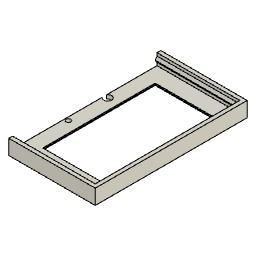
Solar Cell Case Bezel v14 (Autodesk Fusion 360 design; units mm, degrees)
Autodesk Fusion 360 part; units mm, degrees
sketch "Sketch1" plane through (0, 0, 0) normal (0, 0, 1) x (1, 0, 0)
  line L0 (0, 0) -> (44.2, 0)
  line L1 (44.2, 0) -> (44.2, 77.2)
  line L2 (44.2, 77.2) -> (0, 77.2)
  line L3 (0, 77.2) -> (0, 0)
  line L4 (0, 77.2) -> (0, 79.2)
  line L5 (0, 79.2) -> (46.2, 79.2)
  line L6 (46.2, 79.2) -> (46.2, -2)
  line L7 (46.2, -2) -> (0, -2)
  line L8 (0, -2) -> (0, 0)
  dimension "d1" = 44.2
  dimension "d2" = 77.2
  dimension "d3" = 2
  dimension "d4" = 46.2
  dimension "d5" = 2
  constraint horizontal L0
  constraint vertical L1
  constraint horizontal L2
  constraint vertical L3
  constraint coincident L0.start L3.end
  constraint perpendicular L2 L4
  constraint perpendicular L1 L5
  constraint perpendicular L5 L6
  constraint perpendicular L6 L7
  constraint perpendicular L0 L8
  measures "d1" distance of L0.start L0.end
  measures "d2" distance of L0.start L2.end
  measures "d3" distance of L2.end L4.end
  measures "d4" distance of L4.end L5.end
  measures "d5" distance of L0 L7
extrude "Extrude2" add sketch "Sketch1" along normal blind 8 contours L0 L1 L2 L4 L5 L6 L7 L8
extrude "Extrude1" add sketch "Sketch1" along normal blind 2 contours L0 L1 L2 L3
sketch "Sketch2" plane through (0, 0, 0) normal (-1, 0, 0) x (0, -1, 0)
  line L0 (-79.2, 0) -> (2, 0)
  line L1 (-77.2, 2) -> (-77.2, 8)
  line L2 (2, 8) -> (0, 8)
  line L3 (-79.2, 8) -> (-79.2, 0)
  line L4 (2, 0) -> (2, 8)
  line L5 (0, 8) -> (0, 2)
  line L6 (0, 2) -> (-77.2, 2)
  line L7 (-77.2, 8) -> (-79.2, 8)
  line L8 (-77.2, 3.55) -> (-76.2, 5)
  line L9 (-76.2, 5) -> (-77.2, 6.45)
  line L10 (-77.2, 3.55) -> (-77.2, 6.45)
  line L11 (0, 3.55) -> (-1, 5)
  line L12 (-1, 5) -> (0, 6.45)
  line L13 (0, 3.55) -> (0, 6.45)
  dimension "d10" = 5
  dimension "d11" = 2.9
  dimension "d12" = 1.55
  dimension "d13" = 1
  dimension "d14" = 1.45
  dimension "d15" = 1
  constraint coincident L1 L8.start
  constraint coincident L1 L9.end
  constraint parallel L1 L10
  constraint coincident L5 L11.start
  constraint coincident L5 L12.end
  constraint parallel L5 L13
  constraint horizontal L9.end L12.end
  constraint horizontal L8.start L11.start
  constraint horizontal L8.end L11.end
  measures "d11" distance of L8.start L9.end
  measures "d12" distance of L1.end L9.end
  measures "d13" distance of L8.end L10
  measures "d14" vertical distance of L8.end L9.end
  measures "d15" distance of L11.end L13
extrude "Extrude3" add sketch "Sketch2" against normal up to surface (44.2 mm away) contours L1 L8 L9 L10 | L5 L11 L12 L13
hole "Hole1" at (1.75, 28.1, 0) direction (0, 0, 1) diameter 2.5 depth 3 tip angle 118
hole "Hole2" at (1.75, 49.1, 0) direction (0, 0, 1) diameter 4.2 depth 3 tip angle 118
sketch "Sketch3" plane through (0, 0, 2) normal (0, 0, 1) x (-1, 0, 0)
  arc A0 (0, -47.9392) -> (0, -50.2608) centre (-1.75, -49.1) ccw
  line L0 (0, -47.9392) -> (0, 0)
  line L1 (0, 0) -> (-44.2, 0)
  line L2 (-44.2, 0) -> (-44.2, -77.2)
  line L3 (-44.2, -77.2) -> (0, -77.2)
  line L4 (0, -77.2) -> (0, -50.2608)
  circle A1 centre (-1.75, -28.1) radius 1.25
  line L5 (-7.6, -68.6) -> (-38.6, -68.6)
  line L6 (-38.6, -68.6) -> (-38.6, -8.6)
  line L7 (-38.6, -8.6) -> (-7.6, -8.6)
  line L8 (-7.6, -8.6) -> (-7.6, -68.6)
  line L9 (-44.2, 0) -> (-44.2, -77.2)
  line L10 (0, -76.2) -> (-44.2, -76.2)
  line L11 (0, -77.2) -> (0, 0)
  line L12 (-44.2, -77.2) -> (0, -77.2)
  dimension "d33" = 31
  dimension "d34" = 60
  dimension "d35" = 77.2
  dimension "d36" = 44.2
  dimension "d38" = 5.6
  dimension "d40" = 8.6
  constraint horizontal L5
  constraint vertical L6
  constraint horizontal L7
  constraint vertical L8
  measures "d33" distance of L5.start L5.end
  measures "d34" distance of L5.start L7.end
  measures "d35" distance of L1.end L2.end
  measures "d36" distance of L10.start L10.end
  measures "d38" distance of L6 L9
  measures "d40" distance of L5 L12
extrude "Extrude4" cut sketch "Sketch3" against normal blind 3 contours L5 L6 L7 L8
chamfer "Chamfer1" distance 1 angle 55 4 edges at (38.6, 38.6, 0) (23.1, 8.6, 0) (7.6, 38.6, 0) (23.1, 68.6, 0) measured on face at (17.9333, 1.5333, 0) measured on face at (17.9333, 1.5333, 0) measured on face at (17.9333, 1.5333, 0) measured on face at (17.9333, 1.5333, 0)
sketch "Sketch4" plane through (0, 0, 0) normal (0, 0, -1) x (1, 0, 0)
  circle A0 centre (1.75, -28.1) radius 1.25
  arc A1 (0, -50.2608) -> (0, -47.9392) centre (1.75, -49.1) ccw
  line L0 (0, -50.2608) -> (0, -79.2)
  line L1 (0, -79.2) -> (46.2, -79.2)
  line L2 (46.2, -79.2) -> (46.2, 2)
  line L3 (46.2, 2) -> (0, 2)
  line L4 (0, 2) -> (0, -47.9392)
  line L5 (39.6, -7.6) -> (39.6, -69.6)
  line L6 (39.6, -69.6) -> (6.6, -69.6)
  line L7 (6.6, -69.6) -> (6.6, -7.6)
  line L8 (6.6, -7.6) -> (39.6, -7.6)
  line L9 (40.9723, -71.136) -> (8.7716, -71.136) construction
  line L10 (8.7716, -71.136) -> (8.7716, -78.136) construction
  line L11 (8.7716, -78.136) -> (40.9723, -78.136) construction
  line L12 (40.9723, -78.136) -> (40.9723, -71.136) construction
  line L13 (7.9958, -5.6872) -> (37.8791, -5.6872) construction
  line L14 (37.8791, -5.6872) -> (37.8791, 1.3128) construction
  line L15 (37.8791, 1.3128) -> (7.9958, 1.3128) construction
  line L16 (7.9958, 1.3128) -> (7.9958, -5.6872) construction
  text T0 "Ferg Solar" font "Arial" height 7 align ink ink in box 0 x 0 at (40.9623, -71.156) x (-1, 0) y (0, -1) spacing 1 height is em
  text T1 "Go Green" font "Arial" height 7 align ink ink in box 0 x 0 at (8.0058, -5.6672) x (1, 0) y (0, 1) spacing 1 height is em
  constraint perpendicular L9 L10
  constraint parallel L9 L11
  constraint parallel L10 L12
  constraint perpendicular L13 L14
  constraint parallel L13 L15
  constraint parallel L14 L16
extrude "Extrude5" cut sketch "Sketch4" against normal blind 0.5 text T0 T1
sketch "Sketch5" plane through (0, 0, 0) normal (0, 0, -1) x (1, 0, 0)
  line L0 (39.6, -7.6) -> (39.6, -69.6)
  line L1 (39.6, -69.6) -> (6.6, -69.6)
  line L2 (6.6, -69.6) -> (6.6, -7.6)
  line L3 (6.6, -7.6) -> (39.6, -7.6)
  arc A0 (0, -50.2608) -> (0, -47.9392) centre (1.75, -49.1) ccw
  line L4 (0, -50.2608) -> (0, -79.2)
  line L5 (0, -79.2) -> (46.2, -79.2)
  line L6 (46.2, -79.2) -> (46.2, 2)
  line L7 (46.2, 2) -> (0, 2)
  line L8 (0, 2) -> (0, -47.9392)
  circle A1 centre (1.75, -28.1) radius 1.25
  line L9 (11.9912, -4.5495) -> (11.9912, -3.6164)
  line L10 (11.9912, -3.6164) -> (10.5181, -3.6164)
  line L11 (10.5181, -3.6164) -> (10.5181, -3.0285)
  line L12 (10.5181, -3.0285) -> (12.6406, -3.0251)
  line L13 (12.6406, -3.0251) -> (12.6406, -4.8845)
  spline S0 degree 3 poles (12.6406, -4.8845) (12.4792, -5.0053) (12.1657, -5.2398) (11.8065, -5.3953) (11.6323, -5.4707) knots 0 0 0 0 0.06025 0.116987 0.116987 0.116987 0.116987
  spline S1 degree 3 poles (11.6323, -5.4707) (11.4584, -5.528) (11.1118, -5.6422) (10.7474, -5.6589) (10.5659, -5.6672) knots 0 0 0 0 0.054662 0.108889 0.108889 0.108889 0.108889
  spline S2 degree 3 poles (10.5659, -5.6672) (10.3277, -5.6552) (9.861, -5.6316) (9.4336, -5.4432) (9.2244, -5.351) knots 0 0 0 0 0.070895 0.138867 0.138867 0.138867 0.138867
  spline S3 degree 3 poles (9.2244, -5.351) (9.0358, -5.2342) (8.6598, -5.0014) (8.4287, -4.6245) (8.3135, -4.4367) knots 0 0 0 0 0.065553 0.130667 0.130667 0.130667 0.130667
  spline S4 degree 3 poles (8.3135, -4.4367) (8.2238, -4.2287) (8.0399, -3.8022) (8.0174, -3.338) (8.0058, -3.1003) knots 0 0 0 0 0.06739 0.138134 0.138134 0.138134 0.138134
  spline S5 degree 3 poles (8.0058, -3.1003) (8.0181, -2.8616) (8.0423, -2.3889) (8.2225, -1.9514) (8.3118, -1.7348) knots 0 0 0 0 0.071122 0.140843 0.140843 0.140843 0.140843
  spline S6 degree 3 poles (8.3118, -1.7348) (8.4228, -1.5382) (8.6404, -1.153) (9.0106, -0.9114) (9.1919, -0.7932) knots 0 0 0 0 0.066656 0.130584 0.130584 0.130584 0.130584
  spline S7 degree 3 poles (9.1919, -0.7932) (9.3948, -0.7035) (9.8159, -0.5174) (10.2761, -0.4964) (10.5146, -0.4856) knots 0 0 0 0 0.065947 0.136861 0.136861 0.136861 0.136861
  spline S8 degree 3 poles (10.5146, -0.4856) (10.6886, -0.4918) (11.0247, -0.5038) (11.3435, -0.6103) (11.4973, -0.6616) knots 0 0 0 0 0.051926 0.10029 0.10029 0.10029 0.10029
  spline S9 degree 3 poles (11.4973, -0.6616) (11.6338, -0.7236) (11.8956, -0.8425) (12.092, -1.0519) (12.186, -1.1521) knots 0 0 0 0 0.044482 0.085284 0.085284 0.085284 0.085284
  spline S10 degree 3 poles (12.186, -1.1521) (12.2654, -1.2699) (12.4358, -1.5227) (12.5203, -1.8159) (12.5654, -1.9724) knots 0 0 0 0 0.042366 0.090875 0.090875 0.090875 0.090875
  line L14 (12.5654, -1.9724) -> (11.9673, -2.1364)
  spline S11 degree 3 poles (11.9673, -2.1364) (11.9305, -2.0199) (11.8633, -1.8069) (11.742, -1.6197) (11.687, -1.5349) knots 0 0 0 0 0.036444 0.066633 0.066633 0.066633 0.066633
  spline S12 degree 3 poles (11.687, -1.5349) (11.6227, -1.4646) (11.4868, -1.316) (11.3045, -1.2299) (11.2085, -1.1845) knots 0 0 0 0 0.028311 0.059812 0.059812 0.059812 0.059812
  spline S13 degree 3 poles (11.2085, -1.1845) (11.1002, -1.1462) (10.8769, -1.067) (10.64, -1.0577) (10.5181, -1.0529) knots 0 0 0 0 0.034265 0.070644 0.070644 0.070644 0.070644
  spline S14 degree 3 poles (10.5181, -1.0529) (10.3755, -1.0572) (10.1065, -1.0652) (9.8516, -1.151) (9.7319, -1.1914) knots 0 0 0 0 0.042524 0.080213 0.080213 0.080213 0.080213
  spline S15 degree 3 poles (9.7319, -1.1914) (9.6284, -1.2394) (9.4299, -1.3314) (9.2724, -1.4829) (9.197, -1.5554) knots 0 0 0 0 0.033966 0.065103 0.065103 0.065103 0.065103
  spline S16 degree 3 poles (9.197, -1.5554) (9.1332, -1.632) (9.0067, -1.7838) (8.9225, -1.9625) (8.8808, -2.051) knots 0 0 0 0 0.02978 0.059 0.059 0.059 0.059
  spline S17 degree 3 poles (8.8808, -2.051) (8.825, -2.211) (8.7111, -2.5374) (8.6968, -2.883) (8.6894, -3.0593) knots 0 0 0 0 0.050532 0.10313 0.10313 0.10313 0.10313
  spline S18 degree 3 poles (8.6894, -3.0593) (8.696, -3.2671) (8.7081, -3.6547) (8.853, -4.0138) (8.9202, -4.1804) knots 0 0 0 0 0.061793 0.115257 0.115257 0.115257 0.115257
  spline S19 degree 3 poles (8.9202, -4.1804) (9.0052, -4.3208) (9.1741, -4.5994) (9.4533, -4.7671) (9.5918, -4.8503) knots 0 0 0 0 0.04845 0.096145 0.096145 0.096145 0.096145
  spline S20 degree 3 poles (9.5918, -4.8503) (9.7412, -4.9141) (10.0405, -5.0419) (10.3655, -5.06) (10.5283, -5.0691) knots 0 0 0 0 0.048329 0.096832 0.096832 0.096832 0.096832
  spline S21 degree 3 poles (10.5283, -5.0691) (10.6715, -5.062) (10.9598, -5.0477) (11.2321, -4.9516) (11.3691, -4.9033) knots 0 0 0 0 0.042755 0.086105 0.086105 0.086105 0.086105
  spline S22 degree 3 poles (11.3691, -4.9033) (11.4924, -4.8515) (11.7141, -4.7583) (11.906, -4.6137) (11.9912, -4.5495) knots 0 0 0 0 0.039923 0.071805 0.071805 0.071805 0.071805
  line L15 (23.2739, -4.5495) -> (23.2739, -3.6164)
  line L16 (23.2739, -3.6164) -> (21.8008, -3.6164)
  line L17 (21.8008, -3.6164) -> (21.8008, -3.0285)
  line L18 (21.8008, -3.0285) -> (23.9233, -3.0251)
  line L19 (23.9233, -3.0251) -> (23.9233, -4.8845)
  spline S23 degree 3 poles (23.9233, -4.8845) (23.7619, -5.0053) (23.4484, -5.2398) (23.0892, -5.3953) (22.915, -5.4707) knots 0 0 0 0 0.06025 0.116987 0.116987 0.116987 0.116987
  spline S24 degree 3 poles (22.915, -5.4707) (22.7411, -5.528) (22.3946, -5.6422) (22.0301, -5.6589) (21.8486, -5.6672) knots 0 0 0 0 0.054662 0.108889 0.108889 0.108889 0.108889
  spline S25 degree 3 poles (21.8486, -5.6672) (21.6104, -5.6552) (21.1437, -5.6316) (20.7163, -5.4432) (20.5071, -5.351) knots 0 0 0 0 0.070895 0.138867 0.138867 0.138867 0.138867
  spline S26 degree 3 poles (20.5071, -5.351) (20.3185, -5.2342) (19.9425, -5.0014) (19.7114, -4.6245) (19.5962, -4.4367) knots 0 0 0 0 0.065553 0.130667 0.130667 0.130667 0.130667
  spline S27 degree 3 poles (19.5962, -4.4367) (19.5065, -4.2287) (19.3226, -3.8022) (19.3001, -3.338) (19.2886, -3.1003) knots 0 0 0 0 0.06739 0.138134 0.138134 0.138134 0.138134
  spline S28 degree 3 poles (19.2886, -3.1003) (19.3008, -2.8616) (19.325, -2.3889) (19.5053, -1.9514) (19.5945, -1.7348) knots 0 0 0 0 0.071122 0.140843 0.140843 0.140843 0.140843
  spline S29 degree 3 poles (19.5945, -1.7348) (19.7055, -1.5382) (19.9232, -1.153) (20.2934, -0.9114) (20.4746, -0.7932) knots 0 0 0 0 0.066656 0.130584 0.130584 0.130584 0.130584
  spline S30 degree 3 poles (20.4746, -0.7932) (20.6775, -0.7035) (21.0986, -0.5174) (21.5589, -0.4964) (21.7974, -0.4856) knots 0 0 0 0 0.065947 0.136861 0.136861 0.136861 0.136861
  spline S31 degree 3 poles (21.7974, -0.4856) (21.9714, -0.4918) (22.3074, -0.5038) (22.6263, -0.6103) (22.78, -0.6616) knots 0 0 0 0 0.051926 0.10029 0.10029 0.10029 0.10029
  spline S32 degree 3 poles (22.78, -0.6616) (22.9165, -0.7236) (23.1783, -0.8425) (23.3747, -1.0519) (23.4687, -1.1521) knots 0 0 0 0 0.044482 0.085284 0.085284 0.085284 0.085284
  spline S33 degree 3 poles (23.4687, -1.1521) (23.5482, -1.2699) (23.7185, -1.5227) (23.803, -1.8159) (23.8481, -1.9724) knots 0 0 0 0 0.042366 0.090874 0.090874 0.090874 0.090874
  line L20 (23.8481, -1.9724) -> (23.25, -2.1364)
  spline S34 degree 3 poles (23.25, -2.1364) (23.2132, -2.0199) (23.146, -1.8069) (23.0247, -1.6197) (22.9697, -1.5349) knots 0 0 0 0 0.036444 0.066633 0.066633 0.066633 0.066633
  spline S35 degree 3 poles (22.9697, -1.5349) (22.9054, -1.4646) (22.7695, -1.316) (22.5872, -1.2299) (22.4912, -1.1845) knots 0 0 0 0 0.028311 0.059812 0.059812 0.059812 0.059812
  spline S36 degree 3 poles (22.4912, -1.1845) (22.3829, -1.1462) (22.1596, -1.067) (21.9227, -1.0577) (21.8008, -1.0529) knots 0 0 0 0 0.034265 0.070644 0.070644 0.070644 0.070644
  spline S37 degree 3 poles (21.8008, -1.0529) (21.6582, -1.0572) (21.3892, -1.0652) (21.1344, -1.151) (21.0146, -1.1914) knots 0 0 0 0 0.042524 0.080213 0.080213 0.080213 0.080213
  spline S38 degree 3 poles (21.0146, -1.1914) (20.9111, -1.2394) (20.7126, -1.3314) (20.5551, -1.4829) (20.4797, -1.5554) knots 0 0 0 0 0.033966 0.065103 0.065103 0.065103 0.065103
  spline S39 degree 3 poles (20.4797, -1.5554) (20.4159, -1.632) (20.2894, -1.7838) (20.2053, -1.9625) (20.1636, -2.051) knots 0 0 0 0 0.02978 0.059 0.059 0.059 0.059
  spline S40 degree 3 poles (20.1636, -2.051) (20.1077, -2.211) (19.9938, -2.5374) (19.9795, -2.883) (19.9722, -3.0593) knots 0 0 0 0 0.050532 0.10313 0.10313 0.10313 0.10313
  spline S41 degree 3 poles (19.9722, -3.0593) (19.9787, -3.2671) (19.9908, -3.6547) (20.1357, -4.0138) (20.2029, -4.1804) knots 0 0 0 0 0.061793 0.115257 0.115257 0.115257 0.115257
  spline S42 degree 3 poles (20.2029, -4.1804) (20.2879, -4.3208) (20.4568, -4.5994) (20.736, -4.7671) (20.8745, -4.8503) knots 0 0 0 0 0.04845 0.096145 0.096145 0.096145 0.096145
  spline S43 degree 3 poles (20.8745, -4.8503) (21.0239, -4.9141) (21.3232, -5.0419) (21.6482, -5.06) (21.811, -5.0691) knots 0 0 0 0 0.048329 0.096832 0.096832 0.096832 0.096832
  spline S44 degree 3 poles (21.811, -5.0691) (21.9542, -5.062) (22.2425, -5.0477) (22.5148, -4.9516) (22.6518, -4.9033) knots 0 0 0 0 0.042755 0.086104 0.086104 0.086104 0.086104
  spline S45 degree 3 poles (22.6518, -4.9033) (22.7751, -4.8515) (22.9968, -4.7583) (23.1887, -4.6137) (23.2739, -4.5495) knots 0 0 0 0 0.039923 0.071805 0.071805 0.071805 0.071805
  line L21 (25.4307, -3.6814) -> (25.4307, -5.5817)
  line L22 (25.4307, -5.5817) -> (24.8154, -5.5817)
  line L23 (24.8154, -5.5817) -> (24.8154, -1.9519)
  line L24 (24.8154, -1.9519) -> (25.3691, -1.9519)
  line L25 (25.3691, -1.9519) -> (25.3691, -2.5022)
  spline S46 degree 3 poles (25.3691, -2.5022) (25.4308, -2.3903) (25.5357, -2.2002) (25.6949, -2.0534) (25.7605, -1.9929) knots 0 0 0 0 0.037975 0.064591 0.064591 0.064591 0.064591
  spline S47 degree 3 poles (25.7605, -1.9929) (25.8217, -1.957) (25.9438, -1.8854) (26.0849, -1.875) (26.1553, -1.8698) knots 0 0 0 0 0.02098 0.041844 0.041844 0.041844 0.041844
  spline S48 degree 3 poles (26.1553, -1.8698) (26.2618, -1.8797) (26.4865, -1.9004) (26.6839, -2.0103) (26.7876, -2.0681) knots 0 0 0 0 0.031749 0.066919 0.066919 0.066919 0.066919
  line L26 (26.7876, -2.0681) -> (26.5757, -2.6389)
  spline S49 degree 3 poles (26.5757, -2.6389) (26.5021, -2.6) (26.3605, -2.5252) (26.2011, -2.512) (26.1245, -2.5056) knots 0 0 0 0 0.024675 0.047478 0.047478 0.047478 0.047478
  spline S50 degree 3 poles (26.1245, -2.5056) (26.059, -2.5106) (25.9281, -2.5207) (25.8175, -2.5915) (25.7622, -2.6269) knots 0 0 0 0 0.01938 0.038741 0.038741 0.038741 0.038741
  spline S51 degree 3 poles (25.7622, -2.6269) (25.7122, -2.6723) (25.6089, -2.766) (25.559, -2.8964) (25.5332, -2.9636) knots 0 0 0 0 0.019976 0.041227 0.041227 0.041227 0.041227
  spline S52 degree 3 poles (25.5332, -2.9636) (25.5033, -3.0775) (25.4415, -3.3127) (25.4344, -3.5559) (25.4307, -3.6814) knots 0 0 0 0 0.035201 0.072715 0.072715 0.072715 0.072715
  spline S53 degree 3 poles (32.5742, -5.1579) (32.6814, -5.1516) (32.8887, -5.1393) (33.0662, -5.032) (33.1518, -4.9802) knots 0 0 0 0 0.031673 0.061251 0.061251 0.061251 0.061251
  spline S54 degree 3 poles (33.1518, -4.9802) (33.2291, -4.9073) (33.3983, -4.7475) (33.4844, -4.5306) (33.5312, -4.4128) knots 0 0 0 0 0.031501 0.06899 0.06899 0.06899 0.06899
  line L27 (33.5312, -4.4128) -> (34.167, -4.4914)
  spline S55 degree 3 poles (34.167, -4.4914) (34.1086, -4.6649) (33.9955, -5.0005) (33.7355, -5.2403) (33.6099, -5.3562) knots 0 0 0 0 0.053924 0.104353 0.104353 0.104353 0.104353
  spline S56 degree 3 poles (33.6099, -5.3562) (33.4594, -5.4458) (33.1399, -5.6361) (32.7677, -5.6542) (32.5708, -5.6638) knots 0 0 0 0 0.051742 0.109846 0.109846 0.109846 0.109846
  spline S57 degree 3 poles (32.5708, -5.6638) (32.323, -5.6474) (31.8493, -5.616) (31.4827, -5.3163) (31.3078, -5.1733) knots 0 0 0 0 0.072438 0.138524 0.138524 0.138524 0.138524
  spline S58 degree 3 poles (31.3078, -5.1733) (31.172, -4.9837) (30.8784, -4.5742) (30.8543, -4.069) (30.8413, -3.7976) knots 0 0 0 0 0.068525 0.148041 0.148041 0.148041 0.148041
  spline S59 degree 3 poles (30.8413, -3.7976) (30.8541, -3.5172) (30.8778, -2.9967) (31.1756, -2.5717) (31.313, -2.3757) knots 0 0 0 0 0.082198 0.152575 0.152575 0.152575 0.152575
  spline S60 degree 3 poles (31.313, -2.3757) (31.4847, -2.2282) (31.8366, -1.926) (32.2996, -1.8888) (32.5366, -1.8698) knots 0 0 0 0 0.066138 0.13549 0.13549 0.13549 0.13549
  spline S61 degree 3 poles (32.5366, -1.8698) (32.7665, -1.8887) (33.2171, -1.9258) (33.5587, -2.2209) (33.7261, -2.3654) knots 0 0 0 0 0.067288 0.131866 0.131866 0.131866 0.131866
  spline S62 degree 3 poles (33.7261, -2.3654) (33.8604, -2.5576) (34.1519, -2.9746) (34.175, -3.4849) (34.1875, -3.76) knots 0 0 0 0 0.068956 0.149595 0.149595 0.149595 0.149595
  spline S63 degree 3 poles (34.1875, -3.76) (34.1873, -3.7828) (34.1868, -3.8375) (34.1851, -3.8921) (34.1841, -3.924) knots 0 0 0 0 0.006836 0.01641 0.01641 0.01641 0.01641
  line L28 (34.1841, -3.924) -> (31.477, -3.924)
  spline S64 degree 3 poles (31.477, -3.924) (31.4948, -4.1063) (31.5276, -4.4426) (31.725, -4.7152) (31.8154, -4.84) knots 0 0 0 0 0.053778 0.099222 0.099222 0.099222 0.099222
  spline S65 degree 3 poles (31.8154, -4.84) (31.9238, -4.9328) (32.1425, -5.1199) (32.4294, -5.1452) (32.5742, -5.1579) knots 0 0 0 0 0.041673 0.084122 0.084122 0.084122 0.084122
  spline S66 degree 3 poles (35.2714, -73.053) (35.1642, -73.0594) (34.9569, -73.0716) (34.7795, -73.1789) (34.6938, -73.2308) knots 0 0 0 0 0.031673 0.061251 0.061251 0.061251 0.061251
  spline S67 degree 3 poles (34.6938, -73.2308) (34.6165, -73.3037) (34.4473, -73.4634) (34.3612, -73.6803) (34.3144, -73.7981) knots 0 0 0 0 0.031501 0.06899 0.06899 0.06899 0.06899
  line L29 (34.3144, -73.7981) -> (33.6786, -73.7195)
  spline S68 degree 3 poles (33.6786, -73.7195) (33.737, -73.5461) (33.8501, -73.2104) (34.1101, -72.9706) (34.2358, -72.8548) knots 0 0 0 0 0.053924 0.104353 0.104353 0.104353 0.104353
  spline S69 degree 3 poles (34.2358, -72.8548) (34.3862, -72.7651) (34.7057, -72.5748) (35.0779, -72.5567) (35.2748, -72.5472) knots 0 0 0 0 0.051742 0.109846 0.109846 0.109846 0.109846
  spline S70 degree 3 poles (35.2748, -72.5472) (35.5226, -72.5636) (35.9963, -72.595) (36.3629, -72.8947) (36.5378, -73.0376) knots 0 0 0 0 0.072438 0.138524 0.138524 0.138524 0.138524
  spline S71 degree 3 poles (36.5378, -73.0376) (36.6736, -73.2272) (36.9672, -73.6367) (36.9913, -74.142) (37.0043, -74.4134) knots 0 0 0 0 0.068525 0.148041 0.148041 0.148041 0.148041
  spline S72 degree 3 poles (37.0043, -74.4134) (36.9915, -74.6938) (36.9678, -75.2142) (36.67, -75.6392) (36.5326, -75.8352) knots 0 0 0 0 0.082198 0.152575 0.152575 0.152575 0.152575
  spline S73 degree 3 poles (36.5326, -75.8352) (36.3609, -75.9828) (36.009, -76.285) (35.546, -76.3221) (35.309, -76.3411) knots 0 0 0 0 0.066139 0.13549 0.13549 0.13549 0.13549
  spline S74 degree 3 poles (35.309, -76.3411) (35.0791, -76.3222) (34.6285, -76.2852) (34.2869, -75.99) (34.1195, -75.8455) knots 0 0 0 0 0.067288 0.131866 0.131866 0.131866 0.131866
  spline S75 degree 3 poles (34.1195, -75.8455) (33.9852, -75.6533) (33.6937, -75.2363) (33.6706, -74.726) (33.6581, -74.451) knots 0 0 0 0 0.068956 0.149595 0.149595 0.149595 0.149595
  spline S76 degree 3 poles (33.6581, -74.451) (33.6583, -74.4282) (33.6589, -74.3735) (33.6605, -74.3188) (33.6615, -74.2869) knots 0 0 0 0 0.006836 0.01641 0.01641 0.01641 0.01641
  line L30 (33.6615, -74.2869) -> (36.3686, -74.2869)
  spline S77 degree 3 poles (36.3686, -74.2869) (36.3508, -74.1046) (36.318, -73.7684) (36.1206, -73.4958) (36.0302, -73.3709) knots 0 0 0 0 0.053778 0.099222 0.099222 0.099222 0.099222
  spline S78 degree 3 poles (36.0302, -73.3709) (35.9218, -73.2782) (35.7031, -73.091) (35.4162, -73.0658) (35.2714, -73.053) knots 0 0 0 0 0.041673 0.084122 0.084122 0.084122 0.084122
  spline S79 degree 3 poles (29.2524, -71.156) (29.4527, -71.1643) (29.8264, -71.1796) (30.1511, -71.3632) (30.3017, -71.4483) knots 0 0 0 0 0.059157 0.110317 0.110317 0.110317 0.110317
  spline S80 degree 3 poles (30.3017, -71.4483) (30.4176, -71.5626) (30.6618, -71.8035) (30.6789, -72.1476) (30.6879, -72.3284) knots 0 0 0 0 0.047115 0.09929 0.09929 0.09929 0.09929
  line L31 (30.6879, -72.3284) -> (30.0898, -72.2395)
  spline S81 degree 3 poles (30.0898, -72.2395) (30.0741, -72.1555) (30.0451, -71.9993) (29.933, -71.8877) (29.8813, -71.8362) knots 0 0 0 0 0.024955 0.046366 0.046366 0.046366 0.046366
  spline S82 degree 3 poles (29.8813, -71.8362) (29.793, -71.7865) (29.5995, -71.6774) (29.3769, -71.6696) (29.2558, -71.6653) knots 0 0 0 0 0.029967 0.065685 0.065685 0.065685 0.065685
  spline S83 degree 3 poles (29.2558, -71.6653) (29.1267, -71.669) (28.8928, -71.6755) (28.6879, -71.7865) (28.5961, -71.8362) knots 0 0 0 0 0.038094 0.068991 0.068991 0.068991 0.068991
  spline S84 degree 3 poles (28.5961, -71.8362) (28.5246, -71.9002) (28.3775, -72.0317) (28.3142, -72.2187) (28.2817, -72.3147) knots 0 0 0 0 0.028287 0.058133 0.058133 0.058133 0.058133
  spline S85 degree 3 poles (28.2817, -72.3147) (28.2682, -72.4117) (28.2317, -72.6734) (28.2351, -72.9379) (28.2372, -73.1043) knots 0 0 0 0 0.029348 0.079174 0.079174 0.079174 0.079174
  spline S86 degree 3 poles (28.2372, -73.1043) (28.3789, -72.9657) (28.6593, -72.6914) (29.0492, -72.6498) (29.2421, -72.6292) knots 0 0 0 0 0.057625 0.114089 0.114089 0.114089 0.114089
  spline S87 degree 3 poles (29.2421, -72.6292) (29.4754, -72.649) (29.9288, -72.6874) (30.2465, -73.0118) (30.4008, -73.1692) knots 0 0 0 0 0.067753 0.131692 0.131692 0.131692 0.131692
  spline S88 degree 3 poles (30.4008, -73.1692) (30.5204, -73.3617) (30.7668, -73.7582) (30.7959, -74.2246) (30.811, -74.4646) knots 0 0 0 0 0.066881 0.137781 0.137781 0.137781 0.137781
  spline S89 degree 3 poles (30.811, -74.4646) (30.8038, -74.6328) (30.7899, -74.9621) (30.6778, -75.2718) (30.623, -75.4234) knots 0 0 0 0 0.050166 0.09821 0.09821 0.09821 0.09821
  spline S90 degree 3 poles (30.623, -75.4234) (30.555, -75.5603) (30.4228, -75.8265) (30.1906, -76.0118) (30.0778, -76.1018) knots 0 0 0 0 0.045224 0.087981 0.087981 0.087981 0.087981
  spline S91 degree 3 poles (30.0778, -76.1018) (29.9512, -76.1716) (29.6901, -76.3155) (29.3922, -76.3324) (29.2387, -76.3411) knots 0 0 0 0 0.042782 0.088252 0.088252 0.088252 0.088252
  spline S92 degree 3 poles (29.2387, -76.3411) (29.0332, -76.3186) (28.6178, -76.273) (28.3264, -75.9731) (28.1791, -75.8216) knots 0 0 0 0 0.06004 0.121352 0.121352 0.121352 0.121352
  line L32 (28.1791, -75.8216) -> (28.1791, -76.2591)
  line L33 (28.1791, -76.2591) -> (27.6117, -76.2591)
  line L34 (27.6117, -76.2591) -> (27.6117, -73.1214)
  spline S93 degree 3 poles (27.6117, -73.1214) (27.6116, -72.8776) (27.6113, -72.4677) (27.7344, -72.0779) (27.7843, -71.92) knots 0 0 0 0 0.072547 0.121995 0.121995 0.121995 0.121995
  spline S94 degree 3 poles (27.7843, -71.92) (27.8516, -71.8075) (27.989, -71.5777) (28.2155, -71.4344) (28.3312, -71.3611) knots 0 0 0 0 0.038726 0.079169 0.079169 0.079169 0.079169
  spline S95 degree 3 poles (28.3312, -71.3611) (28.4684, -71.3014) (28.7617, -71.1736) (29.0819, -71.1622) (29.2524, -71.156) knots 0 0 0 0 0.044486 0.095118 0.095118 0.095118 0.095118
  spline S96 degree 3 poles (23.8879, -72.742) (24.0322, -72.8155) (24.3172, -72.9606) (24.5126, -73.2136) (24.609, -73.3384) knots 0 0 0 0 0.047942 0.094632 0.094632 0.094632 0.094632
  spline S97 degree 3 poles (24.609, -73.3384) (24.6859, -73.4767) (24.8418, -73.7571) (24.8699, -74.0769) (24.8842, -74.2391) knots 0 0 0 0 0.046883 0.095117 0.095117 0.095117 0.095117
  line L35 (24.8842, -74.2391) -> (24.2587, -74.2937)
  spline S98 degree 3 poles (24.2587, -74.2937) (24.2411, -74.1773) (24.208, -73.9593) (24.1015, -73.7665) (24.0519, -73.6768) knots 0 0 0 0 0.035011 0.065528 0.065528 0.065528 0.065528
  spline S99 degree 3 poles (24.0519, -73.6768) (23.987, -73.5989) (23.848, -73.4322) (23.6521, -73.3376) (23.5478, -73.2872) knots 0 0 0 0 0.030069 0.064372 0.064372 0.064372 0.064372
  spline S100 degree 3 poles (23.5478, -73.2872) (23.4279, -73.2438) (23.1795, -73.1539) (22.9154, -73.1437) (22.7787, -73.1385) knots 0 0 0 0 0.037989 0.078748 0.078748 0.078748 0.078748
  spline S101 degree 3 poles (22.7787, -73.1385) (22.6587, -73.1421) (22.4301, -73.1492) (22.2122, -73.2184) (22.1088, -73.2513) knots 0 0 0 0 0.035829 0.068227 0.068227 0.068227 0.068227
  spline S102 degree 3 poles (22.1088, -73.2513) (22.02, -73.2899) (21.8535, -73.3623) (21.7328, -73.4975) (21.6764, -73.5606) knots 0 0 0 0 0.028648 0.053725 0.053725 0.053725 0.053725
  spline S103 degree 3 poles (21.6764, -73.5606) (21.6351, -73.6271) (21.5532, -73.7588) (21.5408, -73.9132) (21.5346, -73.9895) knots 0 0 0 0 0.023141 0.045765 0.045765 0.045765 0.045765
  spline S104 degree 3 poles (21.5346, -73.9895) (21.5399, -74.0652) (21.5504, -74.2142) (21.6314, -74.3397) (21.6713, -74.4014) knots 0 0 0 0 0.022352 0.044028 0.044028 0.044028 0.044028
  spline S105 degree 3 poles (21.6713, -74.4014) (21.729, -74.4594) (21.8581, -74.5893) (22.0283, -74.6587) (22.1225, -74.6971) knots 0 0 0 0 0.024297 0.054429 0.054429 0.054429 0.054429
  spline S106 degree 3 poles (22.1225, -74.6971) (22.2301, -74.7316) (22.5239, -74.8258) (22.8243, -74.8966) (23.0146, -74.9414) knots 0 0 0 0 0.033906 0.092526 0.092526 0.092526 0.092526
  spline S107 degree 3 poles (23.0146, -74.9414) (23.2124, -74.9887) (23.5433, -75.0678) (23.8561, -75.2007) (23.9818, -75.2542) knots 0 0 0 0 0.060873 0.101811 0.101811 0.101811 0.101811
  spline S108 degree 3 poles (23.9818, -75.2542) (24.092, -75.3178) (24.3011, -75.4386) (24.4475, -75.6302) (24.5168, -75.7207) knots 0 0 0 0 0.037742 0.071604 0.071604 0.071604 0.071604
  spline S109 degree 3 poles (24.5168, -75.7207) (24.5681, -75.8171) (24.6721, -76.0121) (24.6858, -76.2328) (24.6928, -76.3445) knots 0 0 0 0 0.03234 0.065489 0.065489 0.065489 0.065489
  spline S110 degree 3 poles (24.6928, -76.3445) (24.6835, -76.4695) (24.6646, -76.7219) (24.5403, -76.9424) (24.4775, -77.0538) knots 0 0 0 0 0.037093 0.074935 0.074935 0.074935 0.074935
  spline S111 degree 3 poles (24.4775, -77.0538) (24.3952, -77.158) (24.2249, -77.3737) (23.9768, -77.4929) (23.8485, -77.5545) knots 0 0 0 0 0.039284 0.081341 0.081341 0.081341 0.081341
  spline S112 degree 3 poles (23.8485, -77.5545) (23.7043, -77.6043) (23.4066, -77.7072) (23.0916, -77.7192) (22.9291, -77.7254) knots 0 0 0 0 0.045507 0.093974 0.093974 0.093974 0.093974
  spline S113 degree 3 poles (22.9291, -77.7254) (22.7527, -77.7195) (22.416, -77.7081) (22.0979, -77.5982) (21.9464, -77.5459) knots 0 0 0 0 0.052615 0.100393 0.100393 0.100393 0.100393
  spline S114 degree 3 poles (21.9464, -77.5459) (21.8139, -77.4807) (21.5558, -77.3538) (21.3783, -77.1278) (21.2919, -77.0179) knots 0 0 0 0 0.043686 0.085063 0.085063 0.085063 0.085063
  spline S115 degree 3 poles (21.2919, -77.0179) (21.2244, -76.8967) (21.0872, -76.6509) (21.0598, -76.3706) (21.0458, -76.2283) knots 0 0 0 0 0.041128 0.083496 0.083496 0.083496 0.083496
  line L36 (21.0458, -76.2283) -> (21.6816, -76.1805)
  spline S116 degree 3 poles (21.6816, -76.1805) (21.7055, -76.3262) (21.7505, -76.6007) (21.9397, -76.8033) (22.0285, -76.8982) knots 0 0 0 0 0.043187 0.081329 0.081329 0.081329 0.081329
  spline S117 degree 3 poles (22.0285, -76.8982) (22.1476, -76.9688) (22.4154, -77.1275) (22.7281, -77.1361) (22.9018, -77.1409) knots 0 0 0 0 0.040889 0.091965 0.091965 0.091965 0.091965
  spline S118 degree 3 poles (22.9018, -77.1409) (23.0794, -77.1382) (23.3907, -77.1335) (23.662, -76.9844) (23.7785, -76.9205) knots 0 0 0 0 0.052287 0.091608 0.091608 0.091608 0.091608
  spline S119 degree 3 poles (23.7785, -76.9205) (23.8587, -76.8452) (24.0135, -76.7) (24.0406, -76.4901) (24.0536, -76.389) knots 0 0 0 0 0.031888 0.061536 0.061536 0.061536 0.061536
  spline S120 degree 3 poles (24.0536, -76.389) (24.0458, -76.3032) (24.0303, -76.1333) (23.9156, -76.0071) (23.8588, -75.9446) knots 0 0 0 0 0.025087 0.049714 0.049714 0.049714 0.049714
  spline S121 degree 3 poles (23.8588, -75.9446) (23.7453, -75.8814) (23.4334, -75.7075) (23.0824, -75.6341) (22.859, -75.5874) knots 0 0 0 0 0.038808 0.10667 0.10667 0.10667 0.10667
  spline S122 degree 3 poles (22.859, -75.5874) (22.6301, -75.5363) (22.2537, -75.4522) (21.8917, -75.3198) (21.7499, -75.2679) knots 0 0 0 0 0.070266 0.11553 0.11553 0.11553 0.11553
  spline S123 degree 3 poles (21.7499, -75.2679) (21.6164, -75.2001) (21.3662, -75.073) (21.1873, -74.8574) (21.1039, -74.7569) knots 0 0 0 0 0.044366 0.083145 0.083145 0.083145 0.083145
  spline S124 degree 3 poles (21.1039, -74.7569) (21.0431, -74.6485) (20.9189, -74.4271) (20.9034, -74.1736) (20.8954, -74.0442) knots 0 0 0 0 0.036773 0.075111 0.075111 0.075111 0.075111
  spline S125 degree 3 poles (20.8954, -74.0442) (20.9055, -73.9121) (20.9259, -73.644) (21.0576, -73.4095) (21.1244, -73.2906) knots 0 0 0 0 0.039256 0.079622 0.079622 0.079622 0.079622
  spline S126 degree 3 poles (21.1244, -73.2906) (21.2111, -73.1783) (21.3899, -72.9468) (21.649, -72.8105) (21.7824, -72.7403) knots 0 0 0 0 0.042038 0.086674 0.086674 0.086674 0.086674
  spline S127 degree 3 poles (21.7824, -72.7403) (21.9326, -72.683) (22.2435, -72.5644) (22.5761, -72.5508) (22.748, -72.5437) knots 0 0 0 0 0.047911 0.099118 0.099118 0.099118 0.099118
  spline S128 degree 3 poles (22.748, -72.5437) (22.9584, -72.5491) (23.3485, -72.559) (23.7177, -72.6843) (23.8879, -72.742) knots 0 0 0 0 0.062702 0.116289 0.116289 0.116289 0.116289
  line L37 (15.5736, -77.6399) -> (15.5736, -72.6292)
  line L38 (15.5736, -72.6292) -> (16.1889, -72.6292)
  line L39 (16.1889, -72.6292) -> (16.1889, -77.6399)
  line L40 (16.1889, -77.6399) -> (15.5736, -77.6399)
  line L41 (11.4858, -72.6292) -> (12.1283, -72.6292)
  spline S129 degree 3 poles (12.1283, -72.6292) (12.1576, -72.6976) (12.219, -72.8411) (12.2402, -72.9959) (12.2514, -73.0769) knots 0 0 0 0 0.022202 0.046621 0.046621 0.046621 0.046621
  spline S130 degree 3 poles (12.2514, -73.0769) (12.3599, -72.989) (12.5623, -72.8248) (12.7993, -72.7169) (12.9093, -72.6668) knots 0 0 0 0 0.0417 0.077813 0.077813 0.077813 0.077813
  spline S131 degree 3 poles (12.9093, -72.6668) (13.0177, -72.6319) (13.2383, -72.5609) (13.4699, -72.5518) (13.5878, -72.5472) knots 0 0 0 0 0.033976 0.06918 0.06918 0.06918 0.06918
  spline S132 degree 3 poles (13.5878, -72.5472) (13.7699, -72.5544) (14.1046, -72.5678) (14.3811, -72.7543) (14.5072, -72.8394) knots 0 0 0 0 0.053395 0.098176 0.098176 0.098176 0.098176
  spline S133 degree 3 poles (14.5072, -72.8394) (14.6009, -72.9445) (14.7908, -73.1576) (14.8159, -73.4421) (14.8285, -73.5862) knots 0 0 0 0 0.04109 0.083262 0.083262 0.083262 0.083262
  spline S134 degree 3 poles (14.8285, -73.5862) (14.8238, -73.6726) (14.8144, -73.8428) (14.7426, -73.9972) (14.7072, -74.0733) knots 0 0 0 0 0.025686 0.050607 0.050607 0.050607 0.050607
  spline S135 degree 3 poles (14.7072, -74.0733) (14.6641, -74.1428) (14.5793, -74.2797) (14.452, -74.3784) (14.3893, -74.427) knots 0 0 0 0 0.024312 0.047901 0.047901 0.047901 0.047901
  spline S136 degree 3 poles (14.3893, -74.427) (14.321, -74.469) (14.1818, -74.5544) (14.026, -74.6036) (13.9467, -74.6287) knots 0 0 0 0 0.023949 0.048803 0.048803 0.048803 0.048803
  spline S137 degree 3 poles (13.9467, -74.6287) (13.8711, -74.6454) (13.6904, -74.6852) (13.5067, -74.7078) (13.3998, -74.721) knots 0 0 0 0 0.02321 0.055488 0.055488 0.055488 0.055488
  spline S138 degree 3 poles (13.3998, -74.721) (13.1829, -74.7472) (12.812, -74.7921) (12.4521, -74.8916) (12.3027, -74.9329) knots 0 0 0 0 0.065414 0.111879 0.111879 0.111879 0.111879
  spline S139 degree 3 poles (12.3027, -74.9329) (12.3017, -74.9674) (12.3002, -75.0209) (12.2995, -75.0745) (12.2992, -75.0935) knots 0 0 0 0 0.010343 0.016068 0.016068 0.016068 0.016068
  spline S140 degree 3 poles (12.2992, -75.0935) (12.3017, -75.2047) (12.306, -75.4007) (12.4229, -75.5561) (12.4735, -75.6233) knots 0 0 0 0 0.032338 0.05702 0.05702 0.05702 0.05702
  spline S141 degree 3 poles (12.4735, -75.6233) (12.5685, -75.684) (12.781, -75.8196) (13.0342, -75.8275) (13.1742, -75.8318) knots 0 0 0 0 0.03322 0.074311 0.074311 0.074311 0.074311
  spline S142 degree 3 poles (13.1742, -75.8318) (13.3028, -75.8298) (13.5287, -75.8263) (13.7288, -75.7239) (13.8151, -75.6797) knots 0 0 0 0 0.037917 0.06664 0.06664 0.06664 0.06664
  spline S143 degree 3 poles (13.8151, -75.6797) (13.881, -75.613) (14.0303, -75.4618) (14.0885, -75.2563) (14.121, -75.1414) knots 0 0 0 0 0.027698 0.062808 0.062808 0.062808 0.062808
  line L42 (14.121, -75.1414) -> (14.7226, -75.2234)
  spline S144 degree 3 poles (14.7226, -75.2234) (14.6932, -75.3428) (14.6383, -75.5663) (14.5116, -75.7579) (14.4526, -75.8472) knots 0 0 0 0 0.036554 0.068421 0.068421 0.068421 0.068421
  spline S145 degree 3 poles (14.4526, -75.8472) (14.3798, -75.9229) (14.2253, -76.0837) (14.0185, -76.1682) (13.9091, -76.2129) knots 0 0 0 0 0.031148 0.066152 0.066152 0.066152 0.066152
  spline S146 degree 3 poles (13.9091, -76.2129) (13.7821, -76.2503) (13.5133, -76.3293) (13.2331, -76.337) (13.0854, -76.3411) knots 0 0 0 0 0.039553 0.083676 0.083676 0.083676 0.083676
  spline S147 degree 3 poles (13.0854, -76.3411) (12.9439, -76.3387) (12.6872, -76.3344) (12.4407, -76.2635) (12.33, -76.2317) knots 0 0 0 0 0.042215 0.076618 0.076618 0.076618 0.076618
  spline S148 degree 3 poles (12.33, -76.2317) (12.2423, -76.1961) (12.0823, -76.131) (11.9587, -76.0109) (11.9027, -75.9566) knots 0 0 0 0 0.028069 0.05124 0.05124 0.05124 0.05124
  spline S149 degree 3 poles (11.9027, -75.9566) (11.8602, -75.8958) (11.7708, -75.7681) (11.7318, -75.6171) (11.7113, -75.5379) knots 0 0 0 0 0.022064 0.046371 0.046371 0.046371 0.046371
  spline S150 degree 3 poles (11.7113, -75.5379) (11.7025, -75.4645) (11.6797, -75.2761) (11.6803, -75.0863) (11.6806, -74.9705) knots 0 0 0 0 0.022166 0.056867 0.056867 0.056867 0.056867
  line L43 (11.6806, -74.9705) -> (11.6806, -74.1502)
  spline S151 degree 3 poles (11.6806, -74.1502) (11.682, -73.9166) (11.6842, -73.5541) (11.6525, -73.1932) (11.6413, -73.065) knots 0 0 0 0 0.070033 0.10864 0.10864 0.10864 0.10864
  spline S152 degree 3 poles (11.6413, -73.065) (11.6248, -72.9897) (11.5916, -72.8378) (11.5212, -72.6991) (11.4858, -72.6292) knots 0 0 0 0 0.023016 0.046438 0.046438 0.046438 0.046438
  spline S153 degree 3 poles (18.5951, -72.5472) (18.8342, -72.5647) (19.2972, -72.5987) (19.6545, -72.8934) (19.8273, -73.0359) knots 0 0 0 0 0.06999 0.135508 0.135508 0.135508 0.135508
  spline S154 degree 3 poles (19.8273, -73.0359) (19.9641, -73.2279) (20.2629, -73.6473) (20.2852, -74.164) (20.2973, -74.4441) knots 0 0 0 0 0.06928 0.151303 0.151303 0.151303 0.151303
  spline S155 degree 3 poles (20.2973, -74.4441) (20.2833, -74.7497) (20.2575, -75.3116) (19.8999, -75.7416) (19.7367, -75.9378) knots 0 0 0 0 0.088868 0.163454 0.163454 0.163454 0.163454
  spline S156 degree 3 poles (19.7367, -75.9378) (19.5696, -76.0554) (19.2272, -76.2963) (18.8091, -76.3259) (18.5951, -76.3411) knots 0 0 0 0 0.060118 0.123137 0.123137 0.123137 0.123137
  spline S157 degree 3 poles (18.5951, -76.3411) (18.3592, -76.3229) (17.8992, -76.2873) (17.5443, -75.9937) (17.3715, -75.8506) knots 0 0 0 0 0.069114 0.134739 0.134739 0.134739 0.134739
  spline S158 degree 3 poles (17.3715, -75.8506) (17.2331, -75.6631) (16.9368, -75.2618) (16.9105, -74.7618) (16.8964, -74.4954) knots 0 0 0 0 0.068416 0.146443 0.146443 0.146443 0.146443
  spline S159 degree 3 poles (16.8964, -74.4954) (16.9005, -74.284) (16.9079, -73.9038) (17.0455, -73.5502) (17.1066, -73.3931) knots 0 0 0 0 0.062812 0.112991 0.112991 0.112991 0.112991
  spline S160 degree 3 poles (17.1066, -73.3931) (17.1849, -73.2666) (17.3419, -73.0127) (17.5926, -72.8506) (17.7184, -72.7693) knots 0 0 0 0 0.04403 0.088353 0.088353 0.088353 0.088353
  spline S161 degree 3 poles (17.7184, -72.7693) (17.8561, -72.7045) (18.1338, -72.5738) (18.4404, -72.5561) (18.5951, -72.5472) knots 0 0 0 0 0.045183 0.091192 0.091192 0.091192 0.091192
  line L44 (10.1186, -74.5296) -> (10.1186, -72.6292)
  line L45 (10.1186, -72.6292) -> (10.7338, -72.6292)
  line L46 (10.7338, -72.6292) -> (10.7338, -76.2591)
  line L47 (10.7338, -76.2591) -> (10.1801, -76.2591)
  line L48 (10.1801, -76.2591) -> (10.1801, -75.7088)
  spline S162 degree 3 poles (10.1801, -75.7088) (10.1184, -75.8206) (10.0135, -76.0108) (9.8543, -76.1576) (9.7887, -76.2181) knots 0 0 0 0 0.037975 0.064591 0.064591 0.064591 0.064591
  spline S163 degree 3 poles (9.7887, -76.2181) (9.7275, -76.2539) (9.6054, -76.3255) (9.4643, -76.3359) (9.394, -76.3411) knots 0 0 0 0 0.02098 0.041844 0.041844 0.041844 0.041844
  spline S164 degree 3 poles (9.394, -76.3411) (9.2874, -76.3313) (9.0627, -76.3106) (8.8654, -76.2006) (8.7616, -76.1429) knots 0 0 0 0 0.031749 0.066919 0.066919 0.066919 0.066919
  line L49 (8.7616, -76.1429) -> (8.9735, -75.5721)
  spline S165 degree 3 poles (8.9735, -75.5721) (9.0471, -75.6109) (9.1887, -75.6857) (9.3482, -75.699) (9.4247, -75.7054) knots 0 0 0 0 0.024675 0.047478 0.047478 0.047478 0.047478
  spline S166 degree 3 poles (9.4247, -75.7054) (9.4902, -75.7003) (9.6212, -75.6902) (9.7318, -75.6194) (9.787, -75.584) knots 0 0 0 0 0.01938 0.038741 0.038741 0.038741 0.038741
  spline S167 degree 3 poles (9.787, -75.584) (9.8371, -75.5386) (9.9403, -75.4449) (9.9903, -75.3145) (10.016, -75.2474) knots 0 0 0 0 0.019976 0.041227 0.041227 0.041227 0.041227
  spline S168 degree 3 poles (10.016, -75.2474) (10.0459, -75.1335) (10.1077, -74.8982) (10.1149, -74.655) (10.1186, -74.5296) knots 0 0 0 0 0.035201 0.072715 0.072715 0.072715 0.072715
  line L50 (32.2978, -74.5296) -> (32.2978, -72.6292)
  line L51 (32.2978, -72.6292) -> (32.913, -72.6292)
  line L52 (32.913, -72.6292) -> (32.913, -76.2591)
  line L53 (32.913, -76.2591) -> (32.3593, -76.2591)
  line L54 (32.3593, -76.2591) -> (32.3593, -75.7088)
  spline S169 degree 3 poles (32.3593, -75.7088) (32.2976, -75.8206) (32.1927, -76.0108) (32.0335, -76.1576) (31.9679, -76.2181) knots 0 0 0 0 0.037975 0.064591 0.064591 0.064591 0.064591
  spline S170 degree 3 poles (31.9679, -76.2181) (31.9067, -76.2539) (31.7846, -76.3255) (31.6435, -76.3359) (31.5732, -76.3411) knots 0 0 0 0 0.02098 0.041844 0.041844 0.041844 0.041844
  spline S171 degree 3 poles (31.5732, -76.3411) (31.4666, -76.3313) (31.2419, -76.3106) (31.0446, -76.2006) (30.9408, -76.1429) knots 0 0 0 0 0.031749 0.066919 0.066919 0.066919 0.066919
  line L55 (30.9408, -76.1429) -> (31.1527, -75.5721)
  spline S172 degree 3 poles (31.1527, -75.5721) (31.2263, -75.6109) (31.3679, -75.6857) (31.5274, -75.699) (31.6039, -75.7054) knots 0 0 0 0 0.024675 0.047478 0.047478 0.047478 0.047478
  spline S173 degree 3 poles (31.6039, -75.7054) (31.6694, -75.7003) (31.8004, -75.6902) (31.911, -75.6194) (31.9662, -75.584) knots 0 0 0 0 0.019379 0.038741 0.038741 0.038741 0.038741
  spline S174 degree 3 poles (31.9662, -75.584) (32.0163, -75.5386) (32.1195, -75.4449) (32.1695, -75.3145) (32.1952, -75.2474) knots 0 0 0 0 0.019976 0.041227 0.041227 0.041227 0.041227
  spline S175 degree 3 poles (32.1952, -75.2474) (32.2251, -75.1335) (32.2869, -74.8982) (32.2941, -74.655) (32.2978, -74.5296) knots 0 0 0 0 0.035201 0.072715 0.072715 0.072715 0.072715
  line L56 (40.2992, -74.9056) -> (40.2992, -72.6292)
  line L57 (40.2992, -72.6292) -> (40.9623, -72.6292)
  line L58 (40.9623, -72.6292) -> (40.9623, -77.6399)
  line L59 (40.9623, -77.6399) -> (37.5819, -77.6399)
  line L60 (37.5819, -77.6399) -> (37.5819, -77.0486)
  line L61 (37.5819, -77.0486) -> (40.2992, -77.0486)
  line L62 (40.2992, -77.0486) -> (40.2992, -75.4969)
  line L63 (40.2992, -75.4969) -> (37.9477, -75.4969)
  line L64 (37.9477, -75.4969) -> (37.9477, -74.9056)
  line L65 (37.9477, -74.9056) -> (40.2992, -74.9056)
  spline S176 degree 3 poles (28.6811, -5.1579) (28.7883, -5.1516) (28.9956, -5.1393) (29.1731, -5.032) (29.2588, -4.9802) knots 0 0 0 0 0.031673 0.061251 0.061251 0.061251 0.061251
  spline S177 degree 3 poles (29.2588, -4.9802) (29.336, -4.9073) (29.5053, -4.7475) (29.5914, -4.5306) (29.6382, -4.4128) knots 0 0 0 0 0.031501 0.06899 0.06899 0.06899 0.06899
  line L66 (29.6382, -4.4128) -> (30.2739, -4.4914)
  spline S178 degree 3 poles (30.2739, -4.4914) (30.2155, -4.6649) (30.1025, -5.0005) (29.8424, -5.2403) (29.7168, -5.3562) knots 0 0 0 0 0.053924 0.104353 0.104353 0.104353 0.104353
  spline S179 degree 3 poles (29.7168, -5.3562) (29.5663, -5.4458) (29.2469, -5.6361) (28.8746, -5.6542) (28.6777, -5.6638) knots 0 0 0 0 0.051742 0.109846 0.109846 0.109846 0.109846
  spline S180 degree 3 poles (28.6777, -5.6638) (28.43, -5.6474) (27.9562, -5.616) (27.5897, -5.3163) (27.4148, -5.1733) knots 0 0 0 0 0.072438 0.138524 0.138524 0.138524 0.138524
  spline S181 degree 3 poles (27.4148, -5.1733) (27.2789, -4.9837) (26.9854, -4.5742) (26.9612, -4.069) (26.9482, -3.7976) knots 0 0 0 0 0.068525 0.148041 0.148041 0.148041 0.148041
  spline S182 degree 3 poles (26.9482, -3.7976) (26.961, -3.5172) (26.9848, -2.9967) (27.2826, -2.5717) (27.4199, -2.3757) knots 0 0 0 0 0.082198 0.152575 0.152575 0.152575 0.152575
  spline S183 degree 3 poles (27.4199, -2.3757) (27.5917, -2.2282) (27.9435, -1.926) (28.4065, -1.8888) (28.6435, -1.8698) knots 0 0 0 0 0.066139 0.13549 0.13549 0.13549 0.13549
  spline S184 degree 3 poles (28.6435, -1.8698) (28.8735, -1.8887) (29.324, -1.9258) (29.6657, -2.2209) (29.833, -2.3654) knots 0 0 0 0 0.067288 0.131866 0.131866 0.131866 0.131866
  spline S185 degree 3 poles (29.833, -2.3654) (29.9674, -2.5576) (30.2589, -2.9746) (30.282, -3.4849) (30.2944, -3.76) knots 0 0 0 0 0.068956 0.149595 0.149595 0.149595 0.149595
  spline S186 degree 3 poles (30.2944, -3.76) (30.2942, -3.7828) (30.2937, -3.8375) (30.292, -3.8921) (30.291, -3.924) knots 0 0 0 0 0.006836 0.01641 0.01641 0.01641 0.01641
  line L67 (30.291, -3.924) -> (27.584, -3.924)
  spline S187 degree 3 poles (27.584, -3.924) (27.6018, -4.1063) (27.6346, -4.4426) (27.8319, -4.7152) (27.9224, -4.84) knots 0 0 0 0 0.053778 0.099222 0.099222 0.099222 0.099222
  spline S188 degree 3 poles (27.9224, -4.84) (28.0307, -4.9328) (28.2494, -5.1199) (28.5364, -5.1452) (28.6811, -5.1579) knots 0 0 0 0 0.041673 0.084122 0.084122 0.084122 0.084122
  line L68 (35.5547, -3.5993) -> (35.5547, -5.5817)
  line L69 (35.5547, -5.5817) -> (34.9394, -5.5817)
  line L70 (34.9394, -5.5817) -> (34.9394, -1.9519)
  line L71 (34.9394, -1.9519) -> (35.4932, -1.9519)
  line L72 (35.4932, -1.9519) -> (35.4932, -2.468)
  spline S189 degree 3 poles (35.4932, -2.468) (35.6431, -2.2935) (35.9473, -1.9395) (36.4125, -1.8933) (36.6484, -1.8698) knots 0 0 0 0 0.066343 0.134651 0.134651 0.134651 0.134651
  spline S190 degree 3 poles (36.6484, -1.8698) (36.7545, -1.8743) (36.9616, -1.8829) (37.1565, -1.9534) (37.2517, -1.9878) knots 0 0 0 0 0.031626 0.06179 0.06179 0.06179 0.06179
  spline S191 degree 3 poles (37.2517, -1.9878) (37.336, -2.0279) (37.4944, -2.1033) (37.6096, -2.2353) (37.6636, -2.2971) knots 0 0 0 0 0.027647 0.051997 0.051997 0.051997 0.051997
  spline S192 degree 3 poles (37.6636, -2.2971) (37.706, -2.3653) (37.7939, -2.5066) (37.8342, -2.6681) (37.855, -2.7517) knots 0 0 0 0 0.023944 0.049595 0.049595 0.049595 0.049595
  spline S193 degree 3 poles (37.855, -2.7517) (37.8648, -2.8299) (37.8899, -3.0284) (37.8894, -3.2286) (37.8891, -3.3498) knots 0 0 0 0 0.023638 0.059964 0.059964 0.059964 0.059964
  line L73 (37.8891, -3.3498) -> (37.8891, -5.5817)
  line L74 (37.8891, -5.5817) -> (37.2739, -5.5817)
  line L75 (37.2739, -5.5817) -> (37.2739, -3.3737)
  spline S194 degree 3 poles (37.2739, -3.3737) (37.2733, -3.2635) (37.2723, -3.0728) (37.2229, -2.889) (37.2021, -2.8115) knots 0 0 0 0 0.032904 0.056887 0.056887 0.056887 0.056887
  spline S195 degree 3 poles (37.2021, -2.8115) (37.173, -2.7522) (37.1137, -2.6313) (37.0036, -2.5537) (36.9475, -2.5141) knots 0 0 0 0 0.019483 0.039713 0.039713 0.039713 0.039713
  spline S196 degree 3 poles (36.9475, -2.5141) (36.8825, -2.4817) (36.7475, -2.4145) (36.5967, -2.4069) (36.5185, -2.403) knots 0 0 0 0 0.021543 0.044739 0.044739 0.044739 0.044739
  spline S197 degree 3 poles (36.5185, -2.403) (36.3925, -2.413) (36.1429, -2.4328) (35.9403, -2.5798) (35.8401, -2.6525) knots 0 0 0 0 0.037142 0.073551 0.073551 0.073551 0.073551
  spline S198 degree 3 poles (35.8401, -2.6525) (35.7574, -2.7692) (35.5587, -3.0495) (35.5562, -3.3966) (35.5547, -3.5993) knots 0 0 0 0 0.042008 0.100974 0.100974 0.100974 0.100974
  spline S199 degree 3 poles (15.0127, -5.6638) (14.7736, -5.6462) (14.3106, -5.6123) (13.9533, -5.3175) (13.7805, -5.175) knots 0 0 0 0 0.06999 0.135508 0.135508 0.135508 0.135508
  spline S200 degree 3 poles (13.7805, -5.175) (13.6437, -4.983) (13.3449, -4.5637) (13.3226, -4.0469) (13.3105, -3.7668) knots 0 0 0 0 0.06928 0.151303 0.151303 0.151303 0.151303
  spline S201 degree 3 poles (13.3105, -3.7668) (13.3246, -3.4613) (13.3503, -2.8993) (13.7079, -2.4694) (13.8711, -2.2732) knots 0 0 0 0 0.088868 0.163454 0.163454 0.163454 0.163454
  spline S202 degree 3 poles (13.8711, -2.2732) (14.0382, -2.1555) (14.3806, -1.9146) (14.7987, -1.885) (15.0127, -1.8698) knots 0 0 0 0 0.060118 0.123137 0.123137 0.123137 0.123137
  spline S203 degree 3 poles (15.0127, -1.8698) (15.2486, -1.8881) (15.7086, -1.9236) (16.0635, -2.2173) (16.2363, -2.3603) knots 0 0 0 0 0.069114 0.134739 0.134739 0.134739 0.134739
  spline S204 degree 3 poles (16.2363, -2.3603) (16.3747, -2.5478) (16.671, -2.9492) (16.6974, -3.4491) (16.7114, -3.7155) knots 0 0 0 0 0.068416 0.146443 0.146443 0.146443 0.146443
  spline S205 degree 3 poles (16.7114, -3.7155) (16.7073, -3.9269) (16.6999, -4.3072) (16.5623, -4.6608) (16.5012, -4.8178) knots 0 0 0 0 0.062812 0.112991 0.112991 0.112991 0.112991
  spline S206 degree 3 poles (16.5012, -4.8178) (16.4229, -4.9443) (16.2659, -5.1982) (16.0152, -5.3603) (15.8894, -5.4416) knots 0 0 0 0 0.04403 0.088353 0.088353 0.088353 0.088353
  spline S207 degree 3 poles (15.8894, -5.4416) (15.7518, -5.5064) (15.474, -5.6372) (15.1674, -5.6549) (15.0127, -5.6638) knots 0 0 0 0 0.045183 0.091192 0.091192 0.091192 0.091192
equation "d4 = d1 + d3"
equation "d5 = d3"
equation "d12 = ( 6.00 mm - d11 ) / 2"
equation "d14 = d11 / 2"
equation "d15 = d13"
equation "d26 = 30 mm + 0.1 mm"
equation "d38 = ( 44.20 mm - d3 - d33 ) / 2"
equation "d40 = ( 77.20 mm - d34 ) / 2"
